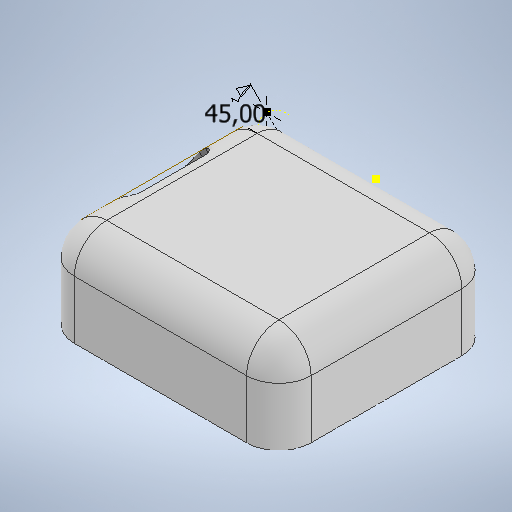
# Autodesk Inventor part: PCB_Deckel
Saved by Autodesk Inventor 2025.2 (Build 292293000, 293)
## iProperties
Created: 2024-11-12
Part Number: PCB_Deckel
Material: Generic
Document SubType Name: Modeling
Designer: matss
Density: 1 g/cm^3
Appearance: Default
Author: matss
Autodesk Inventor part; units mm, degrees
ref_plane "YZ Plane" through (0, 0, 0) normal (1, 0, 0) x (0, 1, 0)
ref_plane "XZ Plane" through (0, 0, 0) normal (0, 1, 0) x (-1, 0, 0)
ref_plane "XY Plane" through (0, 0, 0) normal (0, 0, 1) x (1, 0, 0)
sketch "Sketch1" plane through (0, 0, 0) normal (0, 1, 0) x (-1, 0, 0)
  line L0 (20, 22.5) -> (-20, 22.5)
  line L1 (-25, 17.5) -> (-25, -17.5)
  line L2 (-20, -22.5) -> (20, -22.5)
  line L3 (25, -17.5) -> (25, 17.5)
  arc A0 (25, 17.5) -> (20, 22.5) centre (20, 17.5) ccw
  arc A1 (20, -22.5) -> (25, -17.5) centre (20, -17.5) ccw
  arc A2 (-25, -17.5) -> (-20, -22.5) centre (-20, -17.5) ccw
  arc A3 (-20, 22.5) -> (-25, 17.5) centre (-20, 17.5) ccw
  line L4 (27.5, 17.5) -> (27.5, -17.5)
  arc A4 (20, -25) -> (27.5, -17.5) centre (20, -17.5) ccw
  line L5 (20, -25) -> (-20, -25)
  arc A5 (-27.5, -17.5) -> (-20, -25) centre (-20, -17.5) ccw
  line L6 (-27.5, -17.5) -> (-27.5, 17.5)
  arc A6 (-20, 25) -> (-27.5, 17.5) centre (-20, 17.5) ccw
  line L7 (-20, 25) -> (20, 25)
  arc A7 (27.5, 17.5) -> (20, 25) centre (20, 17.5) ccw
  point P0 (0, 0)
  point P1 (25, 22.5)
  point P2 (25, -22.5)
  point P3 (0, 22.5)
  point P4 (25, 0)
  dimension "d0" = 45
  dimension "d1" = 50
  dimension "d2" = 5
  dimension "d3" = 2.5
  constraints: 16 end point, 16 point on circle, 8 centre point, 8 tangent, 4 parallel, 4 point on line, 3 equal radius, 2 midpoint, 2 perpendicular, 1 horizontal, 1 horizontal alignment, 1 vertical alignment, 7 other
  measures "d0" distance of point (25, -22.5) point (25, 22.5)
  measures "d1" distance between parallel lines of L1 L3
  measures "d2" radius of A0
  measures "d3" distance between parallel lines of L3 L4
extrude "Extrusion1" add sketch "Sketch1" along normal blind 3 contours A0 L3 A1 L2 A2 L1 A3 L0 | L4 A4 L5 A5 L6 A6 L7 A7
extrude "Extrusion2" add sketch "Sketch1" against normal blind 18
fillet "Fillet1" radius 5 8 edges at (23.5355, 0, 21.0355) (0, 0, 22.5) (-23.5355, 0, 21.0355) (-25, 0, 0) (-23.5355, 0, -21.0355) (0, 0, -22.5) (23.5355, 0, -21.0355) (25, 0, 0)
fillet "Fillet2" radius 7.5 8 edges at (-25.3033, 3, -22.8033) (-27.5, 3, 0) (-25.3033, 3, 22.8033) (0, 3, 25) (25.3033, 3, 22.8033) (27.5, 3, 0) (25.3033, 3, -22.8033) (0, 3, -25)
sketch "Sketch2" plane through (20, -18, -25) normal (0, 0, -1) x (-1, 0, 0)
  arc A0 (47.5, 13.5) -> (40, 21) centre (40, 13.5) ccw construction
  line L0 (40, 13.5) -> (45.3033, 18.8033) construction
  line L1 (40, 13.5) -> (47.5, 13.5) construction
  point P0 (20, 18)
  point P1 (45.3033, 18.8033)
  point P2 (45.3033, 18.8033)
  dimension "d10" = 45
  constraints: 4 end point, 2 point on circle, 1 coincident
  measures "d10" angle of L1 L0
ref_plane "Work Plane1" through (-25.3033, 0.8033, -25) normal (-0.7071068, 0.7071068, 0) x (-0.7071068, -0.7071068, 0)
sketch "Sketch3" plane through (-25.3033, 0.8033, -25) normal (-0.7071068, 0.7071068, 0) x (-0.7071068, -0.7071068, 0)
  line L0 (-5.3033, 42.5) -> (-5.3033, 7.5) construction
  line L1 (5.3033, 7.5) -> (5.3033, 42.5) construction
  line L2 (-3.75, 15) -> (3.75, 15)
  line L3 (3.75, 15) -> (3.75, 35)
  line L4 (3.75, 35) -> (-3.75, 35)
  line L5 (-3.75, 35) -> (-3.75, 15)
  line L6 (-5.3033, 25) -> (5.3033, 25) construction
  point P0 (-17.3241, 25)
  point P1 (-3.75, 25)
  point P2 (0, 15)
  point P3 (0, 25)
  dimension "d11" = 7.5
  dimension "d12" = 20
  constraints: 10 end point, 5 midpoint, 2 parallel, 1 horizontal, 1 perpendicular, 1 point on line, 1 vertical alignment
  measures "d11" distance between parallel lines of L3 L5
  measures "d12" distance of L4.end L2.start
extrude "Extrusion3" cut sketch "Sketch3" against normal blind 10
fillet "Fillet3" radius 2.75 4 edges at (-20.5689, 1.3722, -10) (-20.5689, 1.3722, 10) (-26.1204, -3.6829, 10) (-26.1204, -3.6829, -10)
body "Solid1"
